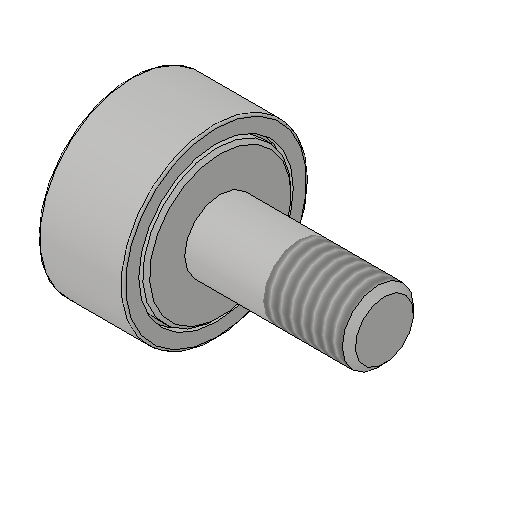
# Autodesk Inventor part: CAM FOLLOWER
Saved by Autodesk Inventor 2022.5 (Build 265521000, 521)
## iProperties
Created: 2023-05-03
Part Number: CAM FOLLOWER
Material: Generic
Catalog Web Link: www.cadenas.de
Description: 3
Vendor: THK
Document SubType Name: Modeling
Designer: psAdmin
Manufacturer: THK
Mass: 8.33717 g
Surface Area: 31.5147 cm^2
Volume: 8.33717 cm^3
Density: 1 g/cm^3
Appearance: PSOLRGB-175-175-175
PSOL_IDENT_0: {$CADENAS_DATA/23d-libs/thk/rotary_series/cam_fllower/popular_type_cf.prj},186 {VTYP=3D},{NB=CF10-1-
PSOL_IDENT_1: CF},{LINA=CF10-1-CF},{NN=Popular Type CF Cam follower},{DATE=17.04.2023 06:52:07},{GEOMDATE=17.09.20
PSOL_IDENT_2: 20 06:17:10},{VERSION=},{LINEID=50},{WBVAR=T,M,SS},{WBNUMERIC=}  {NB=CF10-1-CF},{LINA=CF10-1-CF},{KT=
PSOL_IDENT_3: DUMMY},{SZ=CF10-1},{SZX=CF10-1},{T=},{M=},{SS=},{CNSORDERNO=CF10-1},{SD=10},{D=26},{B=12},{B1=13.0},
PSOL_IDENT_4: {S=M10*1.25},{A=11},{BR=1.500},{RR=8.000},{H=5.000},{I=12.0},{L=36},{D1=4.0},{D2=0},{I1=0},{R=0.3},{
PSOL_IDENT_5: F=15.0},{NDM=10},{KDM=6.466},{T1='', 'with cage', 'V', 'full-roller type'},{C1=0.600}
NB: CF10-1-CF
NN: Popular Type CF Cam follower
NBSYN: $CNSORDERNO.-CF
LINA: CF10-1-CF
CATALOG: THK
SZ: CF10-1
T: with cage
M: No symbol: Carbon steel
SS: without seal
C1: 0.6
SUPPLIER: THK
ARTICLENO: CF10-1-CF
BOMINFO: CF10-1-CF
CREATOR: CADENAS GmbH
MAKER: THK
Detail Description: Purchased products
Title: CF10-1UU
Author: Cadenas PARTsolutions
Revision Number: A
Autodesk Inventor part; units mm, degrees
sketch "Sketch_1" plane through (0, 0, 0) normal (0, 0, 1) x (1, 0, 0)
  line L0 (36, 0) -> (0, 0)
  line L1 (0, 0) -> (0, 9.92)
  line L2 (0, 9.92) -> (0.48, 10.4)
  line L3 (0.48, 10.4) -> (1.6, 10.4)
  line L4 (1.6, 10.4) -> (1.6, 10.8333)
  line L5 (1.6, 10.8333) -> (0.4, 10.8333)
  line L6 (0.4, 10.8333) -> (0.4, 12.7)
  arc A0 (0.7, 13) -> (0.4, 12.7) centre (0.7, 12.7) ccw
  line L7 (0.7, 13) -> (12.1, 13)
  arc A1 (12.4, 12.7) -> (12.1, 13) centre (12.1, 12.7) ccw
  line L8 (12.4, 12.7) -> (12.4, 10.8333)
  line L9 (12.4, 10.8333) -> (11.2, 10.8333)
  line L10 (11.2, 10.8333) -> (11.2, 10.4)
  line L11 (11.2, 10.4) -> (12.52, 10.4)
  line L12 (12.52, 10.4) -> (13, 9.92)
  line L13 (13, 9.92) -> (13, 5)
  line L14 (13, 5) -> (35.08, 5)
  line L15 (35.08, 5) -> (36, 4.08)
  line L16 (36, 4.08) -> (36, 0)
  line L17 (36, 0) -> (0, 0)
  constraints: 36 end point, 4 point on circle, 2 centre point
revolve "Revolution1" add sketch "Sketch_1" angle 360 about axis through (36, 0, 0) along (1, 0, 0)
thread "Thread1" size "M10x1.5" class "6g" standard "ISO Metric profile" length 11.08
sketch "Sketch2" plane through (0, 0, 0) normal (-1, 0, 0) x (0, 0, 1)
  point P0 (0, 0)
hole "Hole1" at (0, 0, 0) direction (1, 0, 0) diameter 4 depth 5.2 tip angle 113.952
sketch "Sketch_5" plane through (0, 0, 0) normal (0, 1, 0) x (-1, 0, 0)
  arc A0 (0, 5.5) -> (-1.375, 2.5) centre (6.4286, 0.7384) ccw
  line L0 (-1.375, 2.5) -> (-1.375, -2.5)
  arc A1 (-1.375, -2.5) -> (0, -5.5) centre (6.4286, -0.7384) ccw
  line L1 (0, -5.5) -> (0, 5.5)
  constraints: 4 end point, 4 point on circle, 2 centre point
extrude "Extrusion1" cut sketch "Sketch_5" along normal mid plane 1.5
ref_plane "IP_dummy_XY" through (0, 0, 0) normal (1, 0, 0) x (0, 0, -1)
ref_plane "IP_dummy_YZ" through (0, 0, 0) normal (0, 0, -1) x (0, 1, 0)
ref_plane "IP_dummy_ZX" through (0, 0, 0) normal (0, 1, 0) x (1, 0, 0)
ref_plane "IP_grease_nipple_XY" through (0, 0, 0) normal (1, 0, 0) x (0, 0, -1)
ref_plane "IP_grease_nipple_YZ" through (0, 0, 0) normal (0, 0, -1) x (0, 1, 0)
ref_plane "IP_grease_nipple_ZX" through (0, 0, 0) normal (0, 1, 0) x (1, 0, 0)
body "Solid1"
